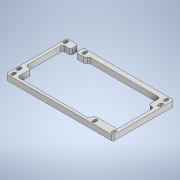
# Autodesk Inventor part: psu_spacer
Saved by Autodesk Inventor 2022 (Build 260153000, 153)
## iProperties
Created: 2021-07-24
Part Number: psu_spacer
Material: Generic
Document SubType Name: Modeling
Designer: gisen
Density: 1 g/cm^3
Appearance: Default
Author: gisen
Autodesk Inventor part; units mm, degrees
ref_plane "YZ Plane" through (0, 0, 0) normal (1, 0, 0) x (0, 1, 0)
ref_plane "XZ Plane" through (0, 0, 0) normal (0, 1, 0) x (-1, 0, 0)
ref_plane "XY Plane" through (0, 0, 0) normal (0, 0, 1) x (1, 0, 0)
sketch "Sketch1" plane through (0, 0, 0) normal (0, 1, 0) x (-1, 0, 0)
  arc A0 (-69, -16.2457) -> (-66, -19.2457) centre (-66, -16.2457) ccw
  line L0 (-64.5, -19.2457) -> (-66, -19.2457)
  arc A1 (-68, -25.7457) -> (-72, -25.7457) centre (-70, -25.7457) ccw
  line L1 (-68, -25.7457) -> (-68, -28.7457)
  line L2 (-72, -28.7457) -> (-72, -25.7457)
  arc A2 (-72, -28.7457) -> (-68, -28.7457) centre (-70, -28.7457) ccw
  line L3 (-61.5, -32.3457) -> (-61.5, -22.2457)
  arc A3 (-66.25, -35.5457) -> (-69.75, -35.5457) centre (-68, -35.5457) ccw
  line L4 (-66.25, -35.5457) -> (-66.25, -38.5457)
  line L5 (-69.75, -38.5457) -> (-69.75, -35.5457)
  arc A4 (-69.75, -38.5457) -> (-66.25, -38.5457) centre (-68, -38.5457) ccw
  arc A5 (-61.5, -22.2457) -> (-64.5, -19.2457) centre (-64.5, -22.2457) ccw
  arc A6 (61.5, 35.0543) -> (58.5, 38.0543) centre (58.5, 35.0543) ccw
  line L6 (61.5, 35.0543) -> (61.5, 21.9543)
  line L7 (66.25, 35.2543) -> (66.25, 38.2543)
  arc A7 (69.75, 38.2543) -> (66.25, 38.2543) centre (68, 38.2543) ccw
  line L8 (69.75, 38.2543) -> (69.75, 35.2543)
  arc A8 (66.25, 35.2543) -> (69.75, 35.2543) centre (68, 35.2543) ccw
  arc A9 (71.75, 28.4543) -> (68.25, 28.4543) centre (70, 28.4543) ccw
  line L9 (71.75, 28.4543) -> (71.75, 25.4543)
  arc A10 (68.25, 25.4543) -> (71.75, 25.4543) centre (70, 25.4543) ccw
  arc A11 (61.5, 21.9543) -> (64.5, 18.9543) centre (64.5, 21.9543) ccw
  line L10 (64.5, 18.9543) -> (66, 18.9543)
  arc A12 (69, 15.9543) -> (66, 18.9543) centre (66, 15.9543) ccw
  line L11 (69, 15.9543) -> (69, -28.7457)
  line L12 (68.25, 25.4543) -> (68.25, 28.4543)
  arc A13 (66, -31.7457) -> (69, -28.7457) centre (66, -28.7457) ccw
  arc A14 (71.75, -35.5457) -> (68.25, -35.5457) centre (70, -35.5457) ccw
  line L13 (71.75, -35.5457) -> (71.75, -38.5457)
  arc A15 (68.25, -38.5457) -> (71.75, -38.5457) centre (70, -38.5457) ccw
  line L14 (68.25, -38.5457) -> (68.25, -35.5457)
  line L15 (66, -31.7457) -> (39.9991, -31.7457)
  arc A16 (45.75, -35.7457) -> (42.25, -35.7457) centre (44, -35.7457) ccw
  arc A17 (39.9991, -31.7457) -> (37.2495, -33.5457) centre (39.9991, -34.7457) ccw
  line L16 (45.75, -35.7457) -> (45.75, -38.7457)
  arc A18 (34.5, -35.3457) -> (37.2495, -33.5457) centre (34.5, -32.3457) ccw
  line L17 (42.25, -38.7457) -> (42.25, -35.7457)
  arc A19 (42.25, -38.7457) -> (45.75, -38.7457) centre (44, -38.7457) ccw
  line L18 (34.5, -35.3457) -> (-58.5, -35.3457)
  arc A20 (-61.5, -32.3457) -> (-58.5, -35.3457) centre (-58.5, -32.3457) ccw
  line L19 (-66, 31.2543) -> (-40.5, 31.2543)
  arc A21 (-71.75, 35.2543) -> (-68.25, 35.2543) centre (-70, 35.2543) ccw
  arc A22 (-68.25, 38.2543) -> (-71.75, 38.2543) centre (-70, 38.2543) ccw
  line L20 (-71.75, 35.2543) -> (-71.75, 38.2543)
  line L21 (-68.25, 38.2543) -> (-68.25, 35.2543)
  line L22 (-69, -16.2457) -> (-69, 28.2543)
  arc A23 (-66, 31.2543) -> (-69, 28.2543) centre (-66, 28.2543) ccw
  line L23 (-45.75, 35.4543) -> (-45.75, 38.4543)
  arc A24 (-42.25, 38.4543) -> (-45.75, 38.4543) centre (-44, 38.4543) ccw
  line L24 (-42.25, 38.4543) -> (-42.25, 35.4543)
  arc A25 (-45.75, 35.4543) -> (-42.25, 35.4543) centre (-44, 35.4543) ccw
  line L25 (-34.5, 38.0543) -> (58.5, 38.0543)
  arc A26 (-34.5, 38.0543) -> (-37.5, 35.0543) centre (-34.5, 35.0543) ccw
  line L26 (-37.5, 34.2543) -> (-37.5, 35.0543)
  arc A27 (-40.5, 31.2543) -> (-37.5, 34.2543) centre (-40.5, 34.2543) ccw
  line L27 (112.7651, 80.6484) -> (-112.7651, 80.6484)
  line L28 (-112.7651, 80.6484) -> (-112.7651, -80.6484)
  line L29 (-112.7651, -80.6484) -> (112.7651, -80.6484)
  line L30 (112.7651, -80.6484) -> (112.7651, 80.6484)
  line L31 (112.7651, 80.6484) -> (-112.7651, -80.6484) construction
  line L32 (-112.7651, 80.6484) -> (112.7651, -80.6484) construction
  point P0 (0, 0)
  dimension "d0" = 1.75
  dimension "d1" = 3
  dimension "d2" = 2
  dimension "d3" = 2
  dimension "d4" = 2.75
  dimension "d5" = 10.25
  dimension "d6" = 26
  dimension "d7" = 109.25
  dimension "d8" = 114
  dimension "d9" = 133.25
  dimension "d10" = 138
  dimension "d11" = 139.75
  dimension "d12" = 140
  dimension "d13" = 140.75
  dimension "d14" = 50.7
  dimension "d15" = 19.1
  dimension "d16" = 54.3
  dimension "d17" = 12.3
  dimension "d18" = 38.2
  dimension "d19" = 9.5
  dimension "d20" = 6.5
  dimension "d21" = 54.5
  dimension "d22" = 57.5
  dimension "d23" = 19.3
  dimension "d24" = 16.3
  dimension "d25" = 54.7
  dimension "d26" = 57.7
  dimension "d27" = 31.7509
  dimension "d28" = 19.5
  dimension "d29" = 16.5
  dimension "d30" = 54.5
  dimension "d31" = 44.7
  dimension "d32" = 137.75
  dimension "d33" = 57.5
  dimension "d34" = 16.3
  dimension "d35" = 139
  dimension "d36" = 19.3
  dimension "d37" = 139
  dimension "d38" = 47.7
  constraints: 66 end point, 56 point on circle, 46 tangent, 28 centre point, 25 equal radius, 21 parallel, 7 perpendicular, 2 midpoint, 1 horizontal
  measures "d0" radius of A9
  measures "d1" radius of A12
  measures "d2" radius of A1
  measures "d3" distance between parallel lines of L8 L9
  measures "d4" distance between parallel lines of L11 L9
  measures "d5" distance between parallel lines of L6 L9
  measures "d6" distance between parallel lines of L9 L16
  measures "d7" distance between parallel lines of L26 L9
  measures "d8" distance between parallel lines of L9 L24
  measures "d9" distance between parallel lines of L3 L9
  measures "d10" distance between parallel lines of L4 L9
  measures "d11" distance between parallel lines of L1 L9
  measures "d12" distance between parallel lines of L9 L21
  measures "d13" distance between parallel lines of L22 L9
  measures "d14" distance between parallel lines of L10 L15
  measures "d15" distance between parallel lines of L25 L10
  measures "d16" distance between parallel lines of L18 L10
  measures "d17" distance between parallel lines of L10 L19
  measures "d18" distance between parallel lines of L0 L10
  measures "d19" distance from line of L9.start L10
  measures "d20" distance from line of L9.end L10
  measures "d21" distance from line of L13.start L10
  measures "d22" distance from line of L13.end L10
  measures "d23" distance from line of L8.start L10
  measures "d24" distance from line of L8.end L10
  measures "d25" distance from line of L16.start L10
  measures "d26" distance from line of L16.end L10
  measures "d27" distance from line of L15.end L9
  measures "d28" distance from line of L24.start L10
  measures "d29" distance from line of L24.end L10
  measures "d30" distance from line of L4.start L10
  measures "d31" distance from line of L1.start L10
  measures "d32" distance from line of A4.centre L8
  measures "d33" distance from line of A4.centre L10
  measures "d34" distance from line of L21.end L10
  measures "d35" distance from line of A22.centre L11
  measures "d36" distance from line of A22.centre L10
  measures "d37" distance from line of A2.centre L11
  measures "d38" distance from line of A2.centre L10
extrude "Extrusion1" add sketch "Sketch1" along normal blind 7.5
sketch "Sketch3" plane through (0, 0, 0) normal (0, -1, 0) x (1, 0, 0)
  line L0 (112.7651, 80.6484) -> (112.7651, -80.6484) projected
  line L1 (-112.7651, 80.6484) -> (112.7651, 80.6484) projected
  line L2 (-112.7651, -80.6484) -> (-112.7651, 80.6484) projected
  line L3 (112.7651, -80.6484) -> (-112.7651, -80.6484) projected
  line L4 (42.25, 38.4543) -> (42.25, 35.4543) projected
  arc A0 (45.75, 38.4543) -> (42.25, 38.4543) centre (44, 38.4543) ccw projected
  line L5 (45.75, 35.4543) -> (45.75, 38.4543) projected
  arc A1 (42.25, 35.4543) -> (45.75, 35.4543) centre (44, 35.4543) ccw projected
  line L6 (71.75, 35.2543) -> (71.75, 38.2543) projected
  arc A2 (68.25, 35.2543) -> (71.75, 35.2543) centre (70, 35.2543) ccw projected
  line L7 (68.25, 38.2543) -> (68.25, 35.2543) projected
  arc A3 (71.75, 38.2543) -> (68.25, 38.2543) centre (70, 38.2543) ccw projected
  line L8 (-71.75, 28.4543) -> (-71.75, 25.4543) projected
  arc A4 (-68.25, 28.4543) -> (-71.75, 28.4543) centre (-70, 28.4543) ccw projected
  line L9 (-68.25, 25.4543) -> (-68.25, 28.4543) projected
  arc A5 (-71.75, 25.4543) -> (-68.25, 25.4543) centre (-70, 25.4543) ccw projected
  line L10 (-69.75, 38.2543) -> (-69.75, 35.2543) projected
  arc A6 (-66.25, 38.2543) -> (-69.75, 38.2543) centre (-68, 38.2543) ccw projected
  line L11 (-66.25, 35.2543) -> (-66.25, 38.2543) projected
  arc A7 (-69.75, 35.2543) -> (-66.25, 35.2543) centre (-68, 35.2543) ccw projected
  line L12 (69.75, -38.5457) -> (69.75, -35.5457) projected
  arc A8 (66.25, -38.5457) -> (69.75, -38.5457) centre (68, -38.5457) ccw projected
  line L13 (66.25, -35.5457) -> (66.25, -38.5457) projected
  arc A9 (69.75, -35.5457) -> (66.25, -35.5457) centre (68, -35.5457) ccw projected
  line L14 (72, -28.7457) -> (72, -25.7457) projected
  arc A10 (68, -28.7457) -> (72, -28.7457) centre (70, -28.7457) ccw projected
  line L15 (68, -25.7457) -> (68, -28.7457) projected
  arc A11 (72, -25.7457) -> (68, -25.7457) centre (70, -25.7457) ccw projected
  line L16 (-68.25, -38.5457) -> (-68.25, -35.5457) projected
  arc A12 (-71.75, -38.5457) -> (-68.25, -38.5457) centre (-70, -38.5457) ccw projected
  line L17 (-71.75, -35.5457) -> (-71.75, -38.5457) projected
  arc A13 (-68.25, -35.5457) -> (-71.75, -35.5457) centre (-70, -35.5457) ccw projected
  line L18 (66, 31.2543) -> (40.5, 31.2543) projected
  arc A14 (69, 28.2543) -> (66, 31.2543) centre (66, 28.2543) ccw projected
  line L19 (69, -16.2457) -> (69, 28.2543) projected
  arc A15 (66, -19.2457) -> (69, -16.2457) centre (66, -16.2457) ccw projected
  line L20 (64.5, -19.2457) -> (66, -19.2457) projected
  arc A16 (64.5, -19.2457) -> (61.5, -22.2457) centre (64.5, -22.2457) ccw projected
  line L21 (61.5, -32.3457) -> (61.5, -22.2457) projected
  arc A17 (58.5, -35.3457) -> (61.5, -32.3457) centre (58.5, -32.3457) ccw projected
  line L22 (-34.5, -35.3457) -> (58.5, -35.3457) projected
  arc A18 (-37.2495, -33.5457) -> (-34.5, -35.3457) centre (-34.5, -32.3457) ccw projected
  arc A19 (-37.2495, -33.5457) -> (-39.9991, -31.7457) centre (-39.9991, -34.7457) ccw projected
  line L23 (-66, -31.7457) -> (-39.9991, -31.7457) projected
  arc A20 (-69, -28.7457) -> (-66, -31.7457) centre (-66, -28.7457) ccw projected
  line L24 (-69, 15.9543) -> (-69, -28.7457) projected
  arc A21 (-66, 18.9543) -> (-69, 15.9543) centre (-66, 15.9543) ccw projected
  line L25 (-64.5, 18.9543) -> (-66, 18.9543) projected
  arc A22 (-64.5, 18.9543) -> (-61.5, 21.9543) centre (-64.5, 21.9543) ccw projected
  line L26 (-61.5, 35.0543) -> (-61.5, 21.9543) projected
  arc A23 (-58.5, 38.0543) -> (-61.5, 35.0543) centre (-58.5, 35.0543) ccw projected
  line L27 (34.5, 38.0543) -> (-58.5, 38.0543) projected
  arc A24 (37.5, 35.0543) -> (34.5, 38.0543) centre (34.5, 35.0543) ccw projected
  line L28 (37.5, 34.2543) -> (37.5, 35.0543) projected
  arc A25 (37.5, 34.2543) -> (40.5, 31.2543) centre (40.5, 34.2543) ccw projected
  line L29 (-45.75, -35.7457) -> (-45.75, -38.7457) projected
  arc A26 (-42.25, -35.7457) -> (-45.75, -35.7457) centre (-44, -35.7457) ccw projected
  line L30 (-42.25, -38.7457) -> (-42.25, -35.7457) projected
  arc A27 (-45.75, -38.7457) -> (-42.25, -38.7457) centre (-44, -38.7457) ccw projected
  line L31 (71.5, -41.9957) -> (-71.25, -41.9957)
  line L32 (-73.25, -39.9957) -> (-73.25, 39.7043)
  line L33 (-71.25, 41.7043) -> (71.5, 41.7043)
  line L34 (73.5, 39.7043) -> (73.5, -39.9957)
  line L35 (73.5, -41.9957) -> (-73.25, 41.7043) construction
  line L36 (-73.25, -41.9957) -> (73.5, 41.7043) construction
  arc A28 (73.5, 39.7043) -> (71.5, 41.7043) centre (71.5, 39.7043) ccw
  arc A29 (71.5, -41.9957) -> (73.5, -39.9957) centre (71.5, -39.9957) ccw
  arc A30 (-73.25, -39.9957) -> (-71.25, -41.9957) centre (-71.25, -39.9957) ccw
  arc A31 (-71.25, 41.7043) -> (-73.25, 39.7043) centre (-71.25, 39.7043) ccw
  point P0 (0.125, -0.1457)
  dimension "d42" = 1.5
  dimension "d43" = 1.5
  dimension "d44" = 1.5
  dimension "d45" = 1.5
  dimension "d46" = 2
  dimension "d47" = 2
  dimension "d48" = 2
  dimension "d49" = 2
  constraints: 12 end point, 8 point on circle, 8 point on line, 8 tangent, 4 centre point, 2 midpoint, 2 parallel, 1 horizontal, 1 perpendicular
  measures "d42" distance between parallel lines of L34 L14
  measures "d43" distance between parallel lines of L8 L32
  measures "d44" distance edge to line of A0 L33
  measures "d45" distance edge to line of A27 L31
  measures "d46" radius of A28
  measures "d47" radius of A29
  measures "d48" radius of A30
  measures "d49" radius of A31
extrude "Extrusion2" cut sketch "Sketch3" against normal up to surface (7.5 mm away) contours L0 L3 L2 L1
sketch "Sketch4" plane through (0, 0, 0) normal (0, -1, 0) x (1, 0, 0)
  arc A0 (-71.25, 41.7043) -> (-73.25, 39.7043) centre (-71.25, 39.7043) ccw projected
  line L0 (-73.25, 39.7043) -> (-73.25, -39.9957) projected
  arc A1 (-73.25, -39.9957) -> (-71.25, -41.9957) centre (-71.25, -39.9957) ccw projected
  line L1 (-71.25, -41.9957) -> (71.5, -41.9957) projected
  arc A2 (71.5, -41.9957) -> (73.5, -39.9957) centre (71.5, -39.9957) ccw projected
  line L2 (73.5, -39.9957) -> (73.5, 39.7043) projected
  arc A3 (73.5, 39.7043) -> (71.5, 41.7043) centre (71.5, 39.7043) ccw projected
  line L3 (71.5, 41.7043) -> (-71.25, 41.7043) projected
  line L4 (42.25, 38.4543) -> (42.25, 35.4543) projected
  arc A4 (45.75, 38.4543) -> (42.25, 38.4543) centre (44, 38.4543) ccw projected
  line L5 (45.75, 35.4543) -> (45.75, 38.4543) projected
  arc A5 (42.25, 35.4543) -> (45.75, 35.4543) centre (44, 35.4543) ccw projected
  line L6 (71.75, 35.2543) -> (71.75, 38.2543) projected
  arc A6 (68.25, 35.2543) -> (71.75, 35.2543) centre (70, 35.2543) ccw projected
  line L7 (68.25, 38.2543) -> (68.25, 35.2543) projected
  arc A7 (71.75, 38.2543) -> (68.25, 38.2543) centre (70, 38.2543) ccw projected
  line L8 (-71.75, 28.4543) -> (-71.75, 25.4543) projected
  arc A8 (-68.25, 28.4543) -> (-71.75, 28.4543) centre (-70, 28.4543) ccw projected
  line L9 (-68.25, 25.4543) -> (-68.25, 28.4543) projected
  arc A9 (-71.75, 25.4543) -> (-68.25, 25.4543) centre (-70, 25.4543) ccw projected
  line L10 (-69.75, 38.2543) -> (-69.75, 35.2543) projected
  arc A10 (-66.25, 38.2543) -> (-69.75, 38.2543) centre (-68, 38.2543) ccw projected
  line L11 (-66.25, 35.2543) -> (-66.25, 38.2543) projected
  arc A11 (-69.75, 35.2543) -> (-66.25, 35.2543) centre (-68, 35.2543) ccw projected
  line L12 (69.75, -38.5457) -> (69.75, -35.5457) projected
  arc A12 (66.25, -38.5457) -> (69.75, -38.5457) centre (68, -38.5457) ccw projected
  line L13 (66.25, -35.5457) -> (66.25, -38.5457) projected
  arc A13 (69.75, -35.5457) -> (66.25, -35.5457) centre (68, -35.5457) ccw projected
  line L14 (72, -28.7457) -> (72, -25.7457) projected
  arc A14 (68, -28.7457) -> (72, -28.7457) centre (70, -28.7457) ccw projected
  line L15 (68, -25.7457) -> (68, -28.7457) projected
  arc A15 (72, -25.7457) -> (68, -25.7457) centre (70, -25.7457) ccw projected
  line L16 (-68.25, -38.5457) -> (-68.25, -35.5457) projected
  arc A16 (-71.75, -38.5457) -> (-68.25, -38.5457) centre (-70, -38.5457) ccw projected
  line L17 (-71.75, -35.5457) -> (-71.75, -38.5457) projected
  arc A17 (-68.25, -35.5457) -> (-71.75, -35.5457) centre (-70, -35.5457) ccw projected
  line L18 (66, 31.2543) -> (40.5, 31.2543) projected
  arc A18 (69, 28.2543) -> (66, 31.2543) centre (66, 28.2543) ccw projected
  line L19 (69, -16.2457) -> (69, 28.2543) projected
  arc A19 (66, -19.2457) -> (69, -16.2457) centre (66, -16.2457) ccw projected
  line L20 (64.5, -19.2457) -> (66, -19.2457) projected
  arc A20 (64.5, -19.2457) -> (61.5, -22.2457) centre (64.5, -22.2457) ccw projected
  line L21 (61.5, -32.3457) -> (61.5, -22.2457) projected
  arc A21 (58.5, -35.3457) -> (61.5, -32.3457) centre (58.5, -32.3457) ccw projected
  line L22 (-34.5, -35.3457) -> (58.5, -35.3457) projected
  arc A22 (-37.2495, -33.5457) -> (-34.5, -35.3457) centre (-34.5, -32.3457) ccw projected
  arc A23 (-37.2495, -33.5457) -> (-39.9991, -31.7457) centre (-39.9991, -34.7457) ccw projected
  line L23 (-66, -31.7457) -> (-39.9991, -31.7457) projected
  arc A24 (-69, -28.7457) -> (-66, -31.7457) centre (-66, -28.7457) ccw projected
  line L24 (-69, 15.9543) -> (-69, -28.7457) projected
  arc A25 (-66, 18.9543) -> (-69, 15.9543) centre (-66, 15.9543) ccw projected
  line L25 (-64.5, 18.9543) -> (-66, 18.9543) projected
  arc A26 (-64.5, 18.9543) -> (-61.5, 21.9543) centre (-64.5, 21.9543) ccw projected
  line L26 (-61.5, 35.0543) -> (-61.5, 21.9543) projected
  arc A27 (-58.5, 38.0543) -> (-61.5, 35.0543) centre (-58.5, 35.0543) ccw projected
  line L27 (34.5, 38.0543) -> (-58.5, 38.0543) projected
  arc A28 (37.5, 35.0543) -> (34.5, 38.0543) centre (34.5, 35.0543) ccw projected
  line L28 (37.5, 34.2543) -> (37.5, 35.0543) projected
  arc A29 (37.5, 34.2543) -> (40.5, 31.2543) centre (40.5, 34.2543) ccw projected
  line L29 (-45.75, -35.7457) -> (-45.75, -38.7457) projected
  arc A30 (-42.25, -35.7457) -> (-45.75, -35.7457) centre (-44, -35.7457) ccw projected
  line L30 (-42.25, -38.7457) -> (-42.25, -35.7457) projected
  arc A31 (-45.75, -38.7457) -> (-42.25, -38.7457) centre (-44, -38.7457) ccw projected
  line L31 (71.5, -41.9957) -> (-71.25, -41.9957) projected
  line L32 (-58, -39.9957) -> (-58, -33.7457)
  line L33 (-50.5, -39.9957) -> (-50.5, -33.7457)
  line L34 (-66, -31.7457) -> (-39.9991, -31.7457) projected
  line L35 (-48.5, -41.9957) -> (-48.4604, -41.9957)
  arc A32 (-50.5, -39.9957) -> (-48.5, -41.9957) centre (-48.5, -39.9957) ccw
  line L36 (-48.5, -31.7457) -> (-48.5, -31.7457)
  line L37 (-60, -31.7457) -> (-59.1147, -31.7457)
  line L38 (-60, -41.9957) -> (-59.4647, -41.9957)
  arc A33 (-48.5, -31.7457) -> (-50.5, -33.7457) centre (-48.5, -33.7457) ccw
  arc A34 (-58, -33.7457) -> (-60, -31.7457) centre (-60, -33.7457) ccw
  arc A35 (-60, -41.9957) -> (-58, -39.9957) centre (-60, -39.9957) ccw
  point P0 (0, 0)
  point P1 (-58, -37.3193)
  point P2 (-58, -41.9957)
  point P3 (-58, -31.7457)
  point P4 (-50.5, -41.9957)
  point P5 (-50.5, -31.7457)
  dimension "d52" = 12
  dimension "d53" = 7.5
  dimension "d54" = 2
  dimension "d55" = 2
  constraints: 16 point on line, 12 end point, 8 point on circle, 8 tangent, 4 centre point, 2 equal radius, 2 perpendicular
  measures "d52" horizontal distance of A16.centre point (-58, -37.319)
  measures "d53" distance from line of point (-58, -37.319) L33
  measures "d54" radius of A32
  measures "d55" radius of A33
extrude "Extrusion3" cut sketch "Sketch4" against normal up to surface (7.5 mm away) contours A35 L32 A34 L23 A33 L33 A32 L1
body "Solid1"
